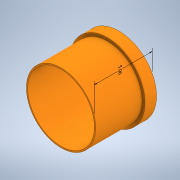
# Autodesk Inventor part: trussTelescopeTubeFront
Saved by Autodesk Inventor 2021.2 (Build 252289000, 289)
## iProperties
Created: 2020-05-22
Part Number: trussTelescopeTubeFront
Material: Aluminum 6061
Document SubType Name: Modeling
Designer: robst
Density: 2.7 g/cm^3
Appearance: Orange
Mass: 3631.37 g
Surface Area: 4474.23 cm^2
Volume: 1344.95 cm^3
Author: robst
Autodesk Inventor part; units mm, degrees
ref_plane "YZ Plane" through (0, 0, 0) normal (1, 0, 0) x (0, 1, 0)
ref_plane "XZ Plane" through (0, 0, 0) normal (0, 1, 0) x (-1, 0, 0)
ref_plane "XY Plane" through (0, 0, 0) normal (0, 0, 1) x (1, 0, 0)
sketch "Sketch1" plane through (0, 0, 0) normal (0, 0, 1) x (1, 0, 0)
  circle A0 centre (0, 0) radius 76.2
  dimension "tubeDiameter" = 152.4
  constraints: 1 centre point, 1 coincident
  measures "tubeDiameter" diameter of A0
extrude "Extrusion1" add sketch "Sketch1" along normal mid plane 438.15
sketch "Sketch2" plane through (0, 0, -219.075) normal (0, 0, -1) x (-1, 0, 0)
  circle A0 centre (0, 0) radius 73.025
  dimension "d6" = 146.05
  constraints: 1 centre point, 1 coincident
  measures "d6" diameter of A0
extrude "Extrusion2" cut sketch "Sketch2" against normal blind 406.4
sketch "Sketch3" plane through (0, 0, 219.075) normal (0, 0, 1) x (1, 0, 0)
  circle A0 centre (0, 0) radius 82.55
  circle A1 centre (0, 0) radius 76.2
  dimension "d9" = 165.1
  constraints: 2 centre point, 2 coincident
  measures "d9" diameter of A0
extrude "Extrusion3" add sketch "Sketch3" against normal blind 25.4
sketch "Sketch4" plane through (0, 0, -219.075) normal (0, 0, -1) x (-1, 0, 0)
  circle A0 centre (0, 0) radius 76.2
  circle A1 centre (0, 0) radius 82.55
  constraints: 2 centre point, 2 coincident
extrude "Extrusion4" add sketch "Sketch4" against normal blind 25.4
sketch "Sketch7" plane through (0, 0, 219.075) normal (0, 0, 1) x (1, 0, 0)
  circle A0 centre (0, 0) radius 82.55 projected
  circle A1 centre (0, 0) radius 82.55
  constraints: 1 centre point, 1 coincident, 1 concentric
extrude "Extrusion6" cut sketch "Sketch7" against normal blind 311.15
body "Solid1"
